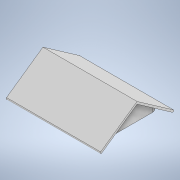
# Autodesk Inventor part: small_top
Saved by Autodesk Inventor 2021 (Build 250183000, 183)
## iProperties
Created: 2021-08-22
Part Number: small_top
Material: Generisch
Document SubType Name: Modeling
Designer: Tilman
Density: 1 g/cm^3
Appearance: Vorgabe
Author: Tilman
Autodesk Inventor part; units mm, degrees
ref_plane "YZ Plane" through (0, 0, 0) normal (1, 0, 0) x (0, 1, 0)
ref_plane "XZ Plane" through (0, 0, 0) normal (0, 1, 0) x (-1, 0, 0)
ref_plane "XY Plane" through (0, 0, 0) normal (0, 0, 1) x (1, 0, 0)
sketch "Skizze1" plane through (0, 0, 0) normal (0, 1, 0) x (-1, 0, 0)
  line L0 (28.5, 24.5) -> (-28.5, 24.5)
  line L1 (-33.5, 19.5) -> (-33.5, -19.5)
  line L2 (-28.5, -24.5) -> (28.5, -24.5)
  line L3 (33.5, -19.5) -> (33.5, 19.5)
  arc A0 (28.5, -24.5) -> (33.5, -19.5) centre (28.5, -19.5) ccw
  arc A1 (-33.5, -19.5) -> (-28.5, -24.5) centre (-28.5, -19.5) ccw
  arc A2 (-28.5, 24.5) -> (-33.5, 19.5) centre (-28.5, 19.5) ccw
  arc A3 (33.5, 19.5) -> (28.5, 24.5) centre (28.5, 19.5) ccw
  point P0 (0, 0)
  point P1 (-33.5, -24.5)
  point P2 (-33.5, 24.5)
  point P3 (33.5, -24.5)
  point P4 (-33.5, 0)
  point P5 (0, -24.5)
  dimension "d0" = 67
  dimension "d1" = 49
  dimension "d2" = 5
  constraints: 8 end point, 8 point on circle, 8 tangent, 6 point on line, 4 centre point, 3 equal radius, 2 midpoint, 2 parallel, 1 horizontal, 1 horizontal alignment, 1 perpendicular, 1 vertical alignment
  measures "d0" distance of point (33.5, -24.5) point (-33.5, -24.5)
  measures "d1" distance of point (-33.5, -24.5) point (-33.5, 24.5)
  measures "d2" radius of A0
extrude "Extrusion1" add sketch "Skizze1" along normal blind 2
sketch "Skizze2" plane through (0, 0, 0) normal (1, 0, 0) x (0, 1, 0)
  line L0 (0, -19.5) -> (0, 19.5) projected
  line L1 (0, 19.5) -> (2, 19.5) projected
  line L2 (2, -19.5) -> (2, 19.5) projected
  line L3 (0, -19.5) -> (2, -19.5) projected
  line L4 (0, -24.5) -> (0, -19.5) projected
  line L5 (0, -19.5) -> (2, -19.5) projected
  line L6 (2, -24.5) -> (2, -19.5) projected
  line L7 (0, -24.5) -> (2, -24.5) projected
  line L8 (0, 19.5) -> (0, 24.5) projected
  line L9 (0, 24.5) -> (2, 24.5) projected
  line L10 (2, 19.5) -> (2, 24.5) projected
  line L11 (0, 19.5) -> (2, 19.5) projected
  line L12 (-1.8519, 30.001) -> (19.1551, 0)
  line L13 (19.1551, 0) -> (-1.8519, -30.001)
  line L14 (-0.5098, 30.9407) -> (21.1551, 0)
  line L15 (21.1551, 0) -> (-0.5098, -30.9407)
  arc A0 (-0.5098, 30.9407) -> (-1.8519, 30.001) centre (-1.1808, 30.4709) ccw
  arc A1 (-1.8519, -30.001) -> (-0.5098, -30.9407) centre (-1.1808, -30.4709) ccw
  line L16 (-2, 38.9986) -> (-2, -40.7887) construction
  point P0 (0, 0)
  point P1 (2, 0)
  dimension "d5" = 35
  dimension "d7" = 2
  dimension "d8" = 2
  constraints: 10 end point, 6 tangent, 4 point on circle, 3 parallel, 2 centre point, 2 horizontal alignment, 2 point on line, 1 equal length, 1 midpoint, 1 vertical alignment
  measures "d5" angle of L2 L12
  measures "d7" distance of L14.end L12.end
  measures "d8" distance from line of point (0, 0) L16
extrude "Extrusion2" add sketch "Skizze2" along normal mid plane 80 contours L13 L12 A0 L14 L15 A1
sketch "Skizze3" plane through (0, 2, 0) normal (0, 1, 0) x (1, 0, 0)
  arc A0 (28.5, -24.5) -> (33.5, -19.5) centre (28.5, -19.5) ccw projected
  line L0 (-28.5, -24.5) -> (28.5, -24.5) projected
  arc A1 (-33.5, -19.5) -> (-28.5, -24.5) centre (-28.5, -19.5) ccw projected
  line L1 (-33.5, 19.5) -> (-33.5, -19.5) projected
  arc A2 (-28.5, 24.5) -> (-33.5, 19.5) centre (-28.5, 19.5) ccw projected
  line L2 (28.5, 24.5) -> (-28.5, 24.5) projected
  arc A3 (33.5, 19.5) -> (28.5, 24.5) centre (28.5, 19.5) ccw projected
  line L3 (33.5, -19.5) -> (33.5, 19.5) projected
  arc A4 (-28.5, 24.5) -> (-33.5, 19.5) centre (-28.5, 19.5) ccw projected
  arc A5 (-33.5, -19.5) -> (-28.5, -24.5) centre (-28.5, -19.5) ccw projected
  line L4 (-28.5, 24.5) -> (-28.5, -24.5)
  line L5 (28.5, 24.5) -> (-28.5, 24.5) projected
  line L6 (-28.5, -24.5) -> (28.5, -24.5) projected
  line L7 (28.5, 24.5) -> (28.5, -24.5)
  point P0 (0, 0)
  constraints: 4 end point, 2 vertical
extrude "Extrusion3" add sketch "Skizze3" along normal up to next contours L7 A3 L3 A0 | A1 L1 A2 L4
sketch "Skizze4" plane through (0, 0, 0) normal (0, -1, 0) x (1, 0, 0)
  arc A0 (33.5, 19.5) -> (28.5, 24.5) centre (28.5, 19.5) ccw projected
  line L0 (-28.5, 24.5) -> (28.5, 24.5) projected
  arc A1 (-28.5, 24.5) -> (-33.5, 19.5) centre (-28.5, 19.5) ccw projected
  line L1 (-33.5, -19.5) -> (-33.5, 19.5) projected
  arc A2 (-33.5, -19.5) -> (-28.5, -24.5) centre (-28.5, -19.5) ccw projected
  line L2 (28.5, -24.5) -> (-28.5, -24.5) projected
  arc A3 (28.5, -24.5) -> (33.5, -19.5) centre (28.5, -19.5) ccw projected
  line L3 (33.5, 19.5) -> (33.5, -19.5) projected
  line L4 (-26, 17) -> (26, 17)
  line L5 (26, 17) -> (26, -17)
  line L6 (26, -17) -> (-26, -17)
  line L7 (-26, -17) -> (-26, 17)
  line L8 (-28.5, 24.5) -> (28.5, 24.5) projected
  point P0 (0, 0)
  point P1 (26, 0)
  point P2 (33.5, 0)
  point P3 (0, 17)
  point P4 (0, 24.5)
  dimension "d13" = 34
  dimension "d14" = 52
  constraints: 8 end point, 4 midpoint, 2 parallel, 1 horizontal, 1 horizontal alignment, 1 perpendicular, 1 vertical alignment
  measures "d13" distance of L6.end L4.start
  measures "d14" distance of L4.start L4.end
extrude "Extrusion4" add sketch "Skizze4" along normal blind 2 contours L4 L5 L6 L7
sketch "Skizze5" plane through (0, -2, 0) normal (0, -1, 0) x (1, 0, 0)
  line L0 (-15, -15) -> (15, -15)
  line L1 (15, -15) -> (15, 15)
  line L2 (15, 15) -> (-15, 15)
  line L3 (-15, 15) -> (-15, -15)
  point P0 (0, 0)
  point P1 (15, 0)
  point P2 (0, 15)
  dimension "d17" = 30
  constraints: 8 end point, 2 midpoint, 2 parallel, 2 perpendicular, 1 horizontal, 1 horizontal alignment, 1 vertical alignment
  measures "d17" distance of L1.end L2.end
extrude "Extrusion5" cut sketch "Skizze5" against normal up to surface (4 mm away)
sketch "Skizze6" plane through (33.5, 0, 19.5) normal (1, 0, 0) x (0, 0, -1)
  line L0 (0, 0) -> (39, 0) projected
  line L1 (39, 0) -> (39, 5.501) projected
  line L2 (19.5, 19.1551) -> (39, 5.501) projected
  line L3 (0, 5.501) -> (19.5, 19.1551) projected
  line L4 (0, 0) -> (0, 5.501) projected
  line L5 (19.5, 18.5447) -> (38.5, 5.2408)
  line L6 (38.5, 5.2408) -> (38.5, 0.5)
  line L7 (38.5, 0.5) -> (0.5, 0.5)
  line L8 (0.5, 0.5) -> (0.5, 5.2408)
  line L9 (0.5, 5.2408) -> (19.5, 18.5447)
  line L10 (0.5, 5.2408) -> (0.2132, 5.6503)
  line L11 (0, 5.501) -> (19.5, 19.1551) projected
  line L12 (38.5, 5.2408) -> (38.7868, 5.6503)
  line L13 (19.5, 19.1551) -> (39, 5.501) projected
  line L14 (17.5, 17.1443) -> (17.2132, 17.5539)
  line L15 (21.5, 17.1443) -> (21.7868, 17.5539)
  point P0 (19.5, 0)
  dimension "d20" = 0.5
  dimension "d23" = 2
  dimension "d24" = 2
  constraints: 18 end point, 6 point on line, 3 perpendicular, 4 other
  measures "d20" distance between parallel lines of L0 L7
  measures "d23" horizontal distance of L5.start L14.start
  measures "d24" horizontal distance of L15.start L5.start
extrude "Extrusion6" cut sketch "Skizze6" against normal through all contours L3 L14 L9 L10 | L12 L5 L15 L2
equation "\"d24\" = d23"
